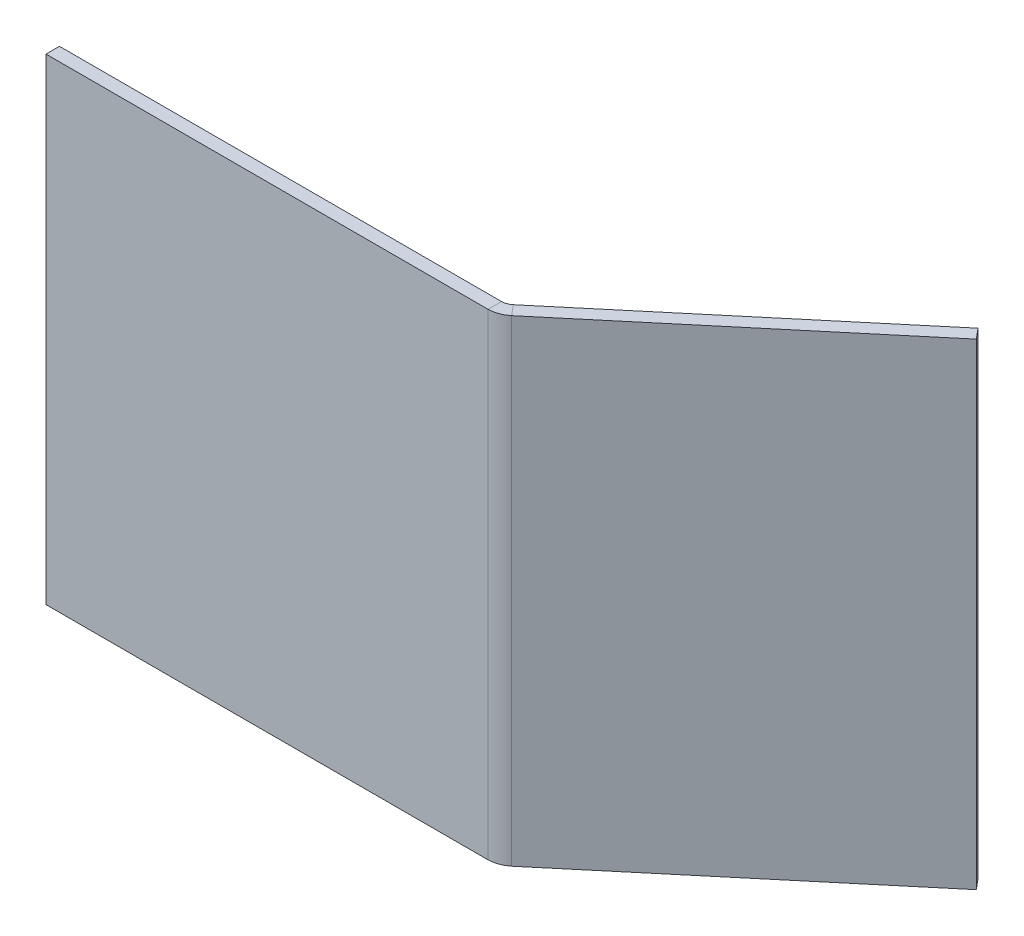
# Autodesk Inventor part: The Law Head
Saved by Autodesk Inventor 2015 SP1 (Build 190203100, 203)
## iProperties
Created: 2015-04-11
Part Number: The Law Head
Material: Aluminum 6061
Document SubType Name: Sheet Metal
Designer: datenney
Density: 2.7 g/cm^3
Sheet Metal Rule: Default
Appearance: Smooth - Black
Author: datenney
Autodesk Inventor part; units mm, degrees
ref_plane "YZ Plane" through (0, 0, 0) normal (1, 0, 0) x (0, 1, 0)
ref_plane "XZ Plane" through (0, 0, 0) normal (0, 1, 0) x (-1, 0, 0)
ref_plane "XY Plane" through (0, 0, 0) normal (0, 0, 1) x (1, 0, 0)
sketch "Sketch1" plane through (0, 0, 0) normal (0, 0, 1) x (1, 0, 0)
  line L0 (-88.9, -53.9686) -> (88.9, -53.9686)
  line L1 (88.9, -53.9686) -> (88.9, 53.9686)
  line L2 (88.9, 53.9686) -> (-88.9, 53.9686)
  line L3 (-88.9, 53.9686) -> (-88.9, -53.9686)
  line L4 (-88.9, -53.9686) -> (88.9, 53.9686) construction
  line L5 (88.9, -53.9686) -> (-88.9, 53.9686) construction
  line L6 (12.7, -53.9686) -> (12.7, 53.9686)
  point P0 (0, 0)
  dimension "d0" = 177.8
  dimension "d1" = 107.9373
  dimension "d2" = 76.2
  constraints: 14 end point, 2 midpoint, 2 parallel, 2 point on line, 1 horizontal, 1 perpendicular, 1 vertical
  measures "d0" distance of L2.end L1.end
  measures "d1" distance of L1.end L0.end
  measures "d2" distance between parallel lines of L1 L6
extrude "Plate1" add sketch "Sketch1" along normal blind 3.048
fold "Fold1" angle 40 bend radius 3.048 thickness 3.048 k factor 0.44 line from (12.7, -53.9686, 0) to (12.7, 53.9686, 0) line at bend centre moving side (1, 0, 0) folds toward (0, 0, -1)
equation "\"d1\" = 1.4165 * d2"
equation "\"d2\" = 0.428571 * d0"
equation "\"d4\" = BendReliefWidth"
equation "\"d5\" = BendReliefDepth"
equation "\"d6\" = MinimumRemnant"
equation "\"d7\" = BendRadius"
equation "\"d9\" = BendRadius"
equation "\"BendRadius\" = Thickness"
equation "\"BendReliefWidth\" = Thickness"
equation "\"BendReliefDepth\" = 0.5 * Thickness"
equation "\"CornerReliefSize\" = 4 * Thickness"
equation "\"MinimumRemnant\" = 2 * Thickness"
equation "\"TransitionRadius\" = BendRadius"
equation "\"JacobiRadiusSize\" = BendRadius"
equation "\"GapSize\" = Thickness"
equation "\"d3\" = BendRadius"
equation "\"Thickness\" = 3.048"
body "Solid1"
